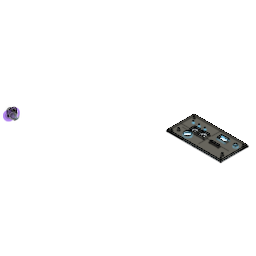
OS backing board brackets v17 (Autodesk Fusion 360 design; units mm, degrees)
Autodesk Fusion 360 part; units mm, degrees
sketch "back content" plane through (0, 0, 0) normal (0, 0, 1) x (1, 0, 0)
  line L0 (174.01, 174.5) -> (274.01, 174.5)
  line L1 (274.01, 174.5) -> (274.01, 124.5)
  line L2 (274.01, 124.5) -> (174.01, 124.5)
  line L3 (174.01, 124.5) -> (174.01, 174.5)
  line L4 (205.01, 145) -> (194.01, 145)
  line L5 (194.01, 145) -> (194.01, 156)
  line L6 (194.01, 156) -> (205.01, 156)
  line L7 (205.01, 156) -> (205.01, 145)
  line L8 (205.01, 145) -> (194.01, 156) construction
  line L9 (194.01, 145) -> (205.01, 156) construction
  line L10 (182.01, 145) -> (246, 145) construction
  line L11 (221.51, 156.5) -> (208.51, 156.5)
  line L12 (208.51, 156.5) -> (208.51, 145)
  line L13 (208.51, 145) -> (221.51, 145)
  line L14 (221.51, 145) -> (221.51, 156.5)
  line L15 (221.51, 156.5) -> (208.51, 145) construction
  line L16 (208.51, 156.5) -> (221.51, 145) construction
  line L17 (248.71, 145) -> (232.71, 145)
  line L18 (232.71, 145) -> (232.71, 148)
  line L19 (232.71, 148) -> (248.71, 148)
  line L20 (248.71, 148) -> (248.71, 145)
  line L21 (248.71, 145) -> (232.71, 148) construction
  line L22 (232.71, 145) -> (248.71, 148) construction
  line L23 (233.51, 158.089) -> (248.51, 158.089)
  line L24 (248.51, 158.089) -> (248.51, 166.689)
  line L25 (248.51, 166.689) -> (233.51, 166.689)
  line L26 (233.51, 166.689) -> (233.51, 158.089)
  circle A0 centre (178.01, 128.5) radius 1
  line L27 (224.01, 174.5) -> (224.01, 124) construction
  line L28 (174.01, 149.5) -> (274.01, 149.5) construction
  circle A1 centre (270.01, 128.5) radius 1
  circle A2 centre (270.01, 170.5) radius 1
  circle A3 centre (178.01, 170.5) radius 1
  circle A4 centre (265.01, 136.3) radius 1.5
  circle A5 centre (183.01, 136.3) radius 1.5
  circle A6 centre (263.3507, 163.0783) radius 3.25
  circle A7 centre (185, 162) radius 1
  circle A8 centre (195.9, 162) radius 1
  circle A9 centre (206.8, 162) radius 1
  circle A10 centre (199.3914, 136.9418) radius 6
  point P0 (199.51, 150.5)
  point P1 (215.01, 150.75)
  point P2 (240.71, 146.5)
  point P3 (195.6, 162)
  point P4 (206.2, 162)
  point P5 (216.8, 162)
  dimension "d381" = 100
  dimension "d382" = 50
  dimension "d5984" = 20.5
  dimension "d5985" = 11
  dimension "d5986" = 11
  dimension "d5988" = 13
  dimension "d5990" = 11.5
  dimension "d5991" = 16
  dimension "d5992" = 3
  dimension "d5998" = 15
  dimension "d5999" = 8.6
  dimension "d6001" = 2
  dimension "d6012" = 46
  dimension "d6013" = 21
  dimension "d6014" = 41
  dimension "d6015" = 3
  dimension "d6040" = 6.5
  dimension "d6041" = 24.5
  dimension "d6043" = 224.01
  dimension "d6044" = 16.7
  dimension "d6045" = 9
  dimension "d6046" = 9.5
  dimension "d6047" = 174.5
  dimension "d6048" = 8.7
  dimension "d6050" = 2
  dimension "d6053" = 10.6
  dimension "d6054" = 0
  dimension "d6057" = 21.8
  dimension "d6058" = 0
  dimension "d6067" = 12
  constraint horizontal L0
  constraint horizontal L2
  constraint vertical L3
  constraint vertical L1
  constraint horizontal L4
  constraint perpendicular L4 L5
  constraint parallel L4 L6
  constraint parallel L5 L7
  constraint coincident L8 P0
  constraint coincident L9 P0
  constraint perpendicular L5 L10
  constraint collinear L4 L10
  constraint horizontal L11
  constraint perpendicular L11 L12
  constraint parallel L11 L13
  constraint parallel L12 L14
  constraint coincident L15 P1
  constraint coincident L16 P1
  constraint collinear L10 L13
  constraint horizontal L17
  constraint perpendicular L17 L18
  constraint parallel L17 L19
  constraint parallel L18 L20
  constraint coincident L21 P2
  constraint coincident L22 P2
  constraint collinear L10 L17
  constraint horizontal L23
  constraint vertical L24
  constraint horizontal L25
  constraint vertical L26
  constraint midpoint L0 L27.start
  constraint perpendicular L0 L27
  constraint midpoint L3 L28.start
  constraint midpoint L1 L28.end
  constraint symmetric A0 L27 A1
  constraint symmetric L28 A1 A2
  constraint symmetric A0 L28 A3
  constraint symmetric L27 A4 A5
  measures "d381" distance of L0.start L0.end
  measures "d382" distance of L0.start L2.end
  measures "d5984" distance of L2 L10
  measures "d5985" distance of L4.end L5.end
  measures "d5986" distance of L5.end L6.end
  measures "d5988" distance of L12.end L13.end
  measures "d5990" distance of L11.start L13.end
  measures "d5991" distance of L18.end L19.end
  measures "d5992" distance of L17.start L19.end
  measures "d5998" distance of L23.start L23.end
  measures "d5999" distance of L23.start L25.end
  measures "d6001" diameter of A0
  measures "d6012" distance of A0.centre L27
  measures "d6013" distance of A0.centre L28
  measures "d6014" distance of L27 A4.centre
  measures "d6015" diameter of A4
  measures "d6040" diameter of A6
  measures "d6041" distance of P0 L27
  measures "d6043" distance of origin L27
  measures "d6044" distance of P2 L27
  measures "d6045" distance of P1 L27
  measures "d6046" distance of L26 L27
  measures "d6047" distance of origin L0
  measures "d6048" distance of L10 A4.centre
  measures "d6050" diameter of A7
  measures "d6067" diameter of A10
sketch "bracket" plane through (0, 0, 0) normal (0, 0, 1) x (1, 0, 0) in component "brackets"
  line L0 (0, 0) -> (11.5, 0)
  line L1 (11.5, 0) -> (11.5, 3.9294)
  line L2 (4, 10.5) -> (0, 10.5)
  line L3 (0, 10.5) -> (0, 0)
  line L4 (6, 3.9294) -> (11.5, 3.9294)
  line L5 (4, 10.5) -> (4, 5.9294)
  arc A0 (4, 5.9294) -> (6, 3.9294) centre (6, 5.9294) ccw
  point P0 (4, 3.9294)
  dimension "d6022" = 11.5
  dimension "d6023" = 10.5
  dimension "d6025" = 2
  dimension "d6049" = 4
  constraint horizontal L0
  constraint vertical L1
  constraint horizontal L2
  constraint vertical L3
  constraint coincident L0.start L3.end
  constraint horizontal L4
  constraint vertical L5
  constraint coincident P0 L4
  constraint coincident P0 L5
  constraint tangent L4 A0
  constraint tangent L5 A0
  measures "d6022" distance of L0.start L0.end
  measures "d6023" distance of L0.start L2.end
  measures "d6025" radius of A0
  measures "d6049" distance of L2.end L2.start
extrude "Extrude2" add sketch "bracket" along normal blind 10 makes body 1 in component "brackets"
sketch "BackingToBracketHole" plane through (0, 0, 0) normal (0, 1, 0) x (1, 0, 0) in component "brackets"
  circle A0 centre (7, -5) radius 1.5
  line L0 (0, 0) -> (0, -10)
  circle A1 centre (7, -5) radius 2.9 construction
  line L1 (6.9779, -8.1753) -> (9.7389, -6.6068)
  line L2 (9.7389, -6.6068) -> (9.761, -3.4314)
  line L3 (9.761, -3.4314) -> (7.0221, -1.8247)
  line L4 (7.0221, -1.8247) -> (4.2611, -3.3932)
  line L5 (4.2611, -3.3932) -> (4.239, -6.5686)
  line L6 (4.239, -6.5686) -> (6.9779, -8.1753)
  point P0 (4, 0)
  point P1 (7, -5)
  dimension "d6028" = 3
  dimension "d6029" = 5
  dimension "d6030" = 7
  dimension "d6061" = 5.8
  constraint concentric A0 A1
  constraint coincident A0.centre A1.centre
  measures "d6028" diameter of A0
  measures "d6029" vertical distance of A0.centre P0
  measures "d6030" distance of A0.centre L0
  measures "d6061" diameter of A1
extrude "Extrude5" cut sketch "BackingToBracketHole" along normal blind 2 from surface at 2.5 bodies 1 in component "brackets"
extrude "Extrude3" cut sketch "BackingToBracketHole" along normal blind 4 contours A0 bodies 1 in component "brackets"
sketch "BracketToPCB" plane through (0, 0, 0) normal (1, 0, 0) x (0, 1, 0) in component "brackets"
  circle A0 centre (4, 5) radius 1.35
  line L0 (10.5, 0) -> (0, 0)
  dimension "d6034" = 2.7
  dimension "d6035" = 5
  dimension "d6036" = 4
  measures "d6034" diameter of A0
  measures "d6035" distance of A0.centre L0
  measures "d6036" horizontal distance of A0.centre L0.end
extrude "Extrude6" cut sketch "BracketToPCB" along normal blind 5 bodies 1 in component "brackets"
extrude "Extrude49" add sketch "back content" along normal blind 3.175 separate body makes body 2
component "brackets" placed x (1, 0, 0) y (0, 1, 0) z (0, 0, 1) at (0, 0, 0)
equation "platformMountHoles = 3 mm"
equation "pcbMountHoles = 2 mm"
equation "b_Length = 150.00 mm" comment "Length (mm)"
equation "b_Depth = 120.00 mm" comment "Depth (mm)"
equation "b_Height = 65.00 mm" comment "Height (mm)"
equation "b_Thickness = 3.175 mm" comment "Thickness (mm)"
equation "b_Tool_diameter = 2.01 mm" comment "Tool Diameter (mm)"
equation "b_Tooth_width = 10.00 mm" comment "Target Tooth Width (mm)"
equation "b_Kerf = -0.16 mm" comment "Kerf (mm)- can be negative"
equation "b_Delta_from_bottom = -0.10 mm" comment "Additional fine adjustment of bone centers from bottom of holes(mm)- positive makes smaller bottom indents"
equation "b_Stock_x_dimension = 304.80 mm" comment "Stock X Dimension *"
equation "b_Stock_y_dimension = 609.60 mm" comment "Stock Y Dimension"
equation "b_Repeats_l_tmp = -1.00 mm" comment "temp hidden"
equation "Version_info = 0 mm" comment "1.2.0 LENGTH 150.0 DEPTH 120.0 HEIGHT 65.0 THICKNESS 3.175 TOOL_DIAMETER 2.01 TOOTH_WIDTH 10.0 KERF -0.16 DELTA_FROM_BOTTOM -0.1 STOCK_X_DIMENSION 304.8 STOCK_Y_DIMENSION 609.6 COMPONENT  REPEATS_L_TMP -1 CREATE_COMPONENTS False CREATE_BODIES 1 CREATE_EMPTY_CONTENTS False CREATE_CONSTRAINTS True CLEAR_PREVIOUSLY_GENERATED_ITEMS True JUST_CLEAR_PREVIOUSLY_GENERATED_ITEMS False CREATE_MANUFACTURING False JUST_CREATE_MANUFACTURING False DEBUG_JUST_ONE_PART False MANUAL_LAYOUT  LASER False JUST_BUILD_TEST False DEBUG True"
equation "shaftCenterToCenter = 34 mm"
equation "shaftCenterToMountingHoles = 15.5 mm"
equation "ballBearingHoleDiam = 12.8 mm"
equation "ballBearingCenterToCenterHoriz = 55 mm"
equation "ballBearingCenterToCenterVert = 40 mm"
equation "Dlc32Length = 82 mm"
equation "d6001 = pcbMountHoles"
equation "d6050 = pcbMountHoles"
equation "d6059 = b_Thickness"
named bodies: "bracket", "backingBoard"
